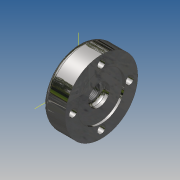
# Autodesk Inventor part: Zylinderkopf_ra8846s
Saved by Autodesk Inventor 2021 (Build 250183000, 183)
## iProperties
Created: 2020-12-15
Part Number: Zylinderkopf_ra8846s
Material: Stahl, Guss
Document SubType Name: Modeling
Designer: Ricardo
Density: 8.06158 g/cm^3
Appearance: Halbpoliert
Mass: 31 g
Surface Area: 22.8629 cm^2
Volume: 3.8454 cm^3
Author: Sander
Revision Number: Rev00
Autodesk Inventor part; units mm, degrees
ref_plane "YZ-Ebene" through (0, 0, 0) normal (1, 0, 0) x (0, 1, 0)
ref_plane "XZ-Ebene" through (0, 0, 0) normal (0, 1, 0) x (-1, 0, 0)
ref_plane "XY-Ebene" through (0, 0, 0) normal (0, 0, 1) x (1, 0, 0)
sketch "Skizze1" plane through (0, 0, 0) normal (0, 0, 1) x (1, 0, 0)
  line L0 (-2.1971, 0) -> (10.2828, 0) projected
  line L1 (0, -2.7828) -> (0, 16.6971) projected
  line L2 (0, 5) -> (1.2, 5)
  line L3 (1.2, 5) -> (1.2, 2.75)
  line L4 (1.2, 2.75) -> (5.2, 2.75)
  arc A0 (6.4, 3.95) -> (5.2, 2.75) centre (6.4, 2.75) ccw
  line L5 (6.4, 3.95) -> (7.6, 3.95)
  line L6 (7.6, 3.95) -> (7.6, 8.75)
  line L7 (7.6, 8.75) -> (8.5, 8.75)
  line L8 (8.5, 8.75) -> (8.5, 13.5)
  line L9 (8.5, 13.5) -> (2, 13.5)
  arc A1 (2, 13.5) -> (0, 11.5) centre (2, 11.5) ccw
  line L10 (0, 11.5) -> (0, 5)
  point P0 (0, 0)
  dimension "d6" = 2.75
  dimension "d7" = 5
  dimension "d8" = 8.75
  dimension "d9" = 13.5
  dimension "d10" = 1.2
  dimension "d11" = 2.4
  dimension "d12" = 0.9
  dimension "d13" = 1.2
  dimension "d14" = 2
  dimension "d15" = 8.5
  constraints: 18 end point, 5 perpendicular, 4 point on circle, 3 point on line, 3 tangent, 2 centre point, 2 horizontal, 1 collinear, 1 vertical
  measures "d6" distance from line of L0 L3.end
  measures "d7" distance from line of L0 L2.start
  measures "d8" distance from line of L0 L7.end
  measures "d9" distance from line of L0 L9.end
  measures "d10" distance of L2.start L2.end
  measures "d11" horizontal distance of L5.end L4.end
  measures "d12" distance of L6.end L7.end
  measures "d13" radius of A0
  measures "d14" radius of A1
  measures "d15" horizontal distance of L8.end L10.start
revolve "Umdrehung1" add sketch "Skizze1" angle 360 about axis through (-10, 0, 0) along (1, 0, 0)
sketch "Skizze2" plane through (0, 0, 0) normal (-1, 0, 0) x (0, 0, 1)
  circle A0 centre (0, 0) radius 5 projected
  line L0 (-18.9, 0) -> (18.9, 0) projected
  circle A1 centre (0, 0) radius 5 projected
  circle A2 centre (0, 0) radius 11.5 projected
  point P0 (10.5, 0)
  dimension "d18" = 10.5
  constraints: 1 point on line
  measures "d18" distance of A0.centre point (10.5, 0)
hole "Bohrung1" at (0, 0, 10.5) direction (1, 0, 0) diameter 3 end through all counterbore diameter 5.5 counterbore depth 3
pattern_circular "Runde Anordnung1" count 4 over 360 about axis through (3.2, 0, 0) along (-1, 0, 0) of "Bohrung1"
thread "Gewinde1" size "M6x0.5" class "6H" standard "ISO Metric profile" length 7
